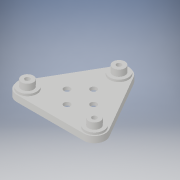
# Autodesk Inventor part: PlanetaryHolderTop
Saved by Autodesk Inventor 2018.3 (Build 223284000, 284)
## iProperties
Created: 2018-07-08
Part Number: PlanetaryHolderTop
Material: Generisch
Document SubType Name: Modeling
Designer: JochenAlt
Density: 1 g/cm^3
Appearance: Vorgabe
Author: JochenAlt
Autodesk Inventor part; units mm, degrees
ref_plane "YZ Plane" through (0, 0, 0) normal (1, 0, 0) x (0, 1, 0)
ref_plane "XZ Plane" through (0, 0, 0) normal (0, 1, 0) x (-1, 0, 0)
ref_plane "XY Plane" through (0, 0, 0) normal (0, 0, 1) x (1, 0, 0)
sketch "Skizze1" plane through (0, 0, 0) normal (0, 0, 1) x (1, 0, 0)
  circle A0 centre (0, 0) radius 18.538 construction
  circle A1 centre (0, 0) radius 9.75
  circle A2 centre (0, 18.538) radius 1.15
  line L0 (0, 0) -> (-16.0544, -9.269) construction
  line L1 (0, 32.8502) -> (0, -27.1027) construction
  line L2 (-31.8422, 0) -> (31.8422, 0) construction
  circle A3 centre (0, 0) radius 6.35 construction
  circle A4 centre (0, 6.35) radius 1.5
  circle A5 centre (0, -6.35) radius 1.5
  circle A6 centre (6.35, 0) radius 1.5
  circle A7 centre (-6.35, 0) radius 1.5
  arc A8 (0, 23.688) -> (-4.46, 21.113) centre (0, 18.538) ccw
  circle A9 centre (16.0544, -9.269) radius 1.15
  arc A10 (16.0544, -14.419) -> (20.5144, -6.694) centre (16.0544, -9.269) ccw
  circle A11 centre (-16.0544, -9.269) radius 1.15
  arc A12 (-20.5144, -6.694) -> (-16.0544, -14.419) centre (-16.0544, -9.269) ccw
  circle A13 centre (0, 18.538) radius 2.85
  circle A14 centre (16.0544, -9.269) radius 2.85
  circle A15 centre (-16.0544, -9.269) radius 2.85
  circle A16 centre (0, 18.538) radius 4.5
  circle A17 centre (16.0544, -9.269) radius 4.5
  circle A18 centre (-16.0544, -9.269) radius 4.5
  line L3 (-4.46, 21.113) -> (-20.5144, -6.694)
  line L4 (-16.0544, -14.419) -> (16.0544, -14.419)
  line L5 (4.46, 21.113) -> (20.5144, -6.694)
  arc A19 (4.46, 21.113) -> (0, 23.688) centre (0, 18.538) ccw
  circle A20 centre (0, 18.538) radius 2.1 construction
  line L6 (1.2124, 20.638) -> (2.4249, 18.538)
  line L7 (2.4249, 18.538) -> (1.2124, 16.438)
  line L8 (1.2124, 16.438) -> (-1.2124, 16.438)
  line L9 (-1.2124, 16.438) -> (-2.4249, 18.538)
  line L10 (-2.4249, 18.538) -> (-1.2124, 20.638)
  line L11 (-1.2124, 20.638) -> (1.2124, 20.638)
  circle A21 centre (-16.0544, -9.269) radius 2.1 construction
  circle A22 centre (16.0544, -9.269) radius 2.1 construction
  line L12 (-17.2654, -11.3698) -> (-18.4792, -9.2707)
  line L13 (-18.4792, -9.2707) -> (-17.2683, -7.1698)
  line L14 (-17.2683, -7.1698) -> (-14.8434, -7.1682)
  line L15 (-14.8434, -7.1682) -> (-13.6295, -9.2673)
  line L16 (-13.6295, -9.2673) -> (-14.8405, -11.3682)
  line L17 (-14.8405, -11.3682) -> (-17.2654, -11.3698)
  line L18 (15.1602, -11.523) -> (13.6553, -9.6216)
  line L19 (13.6553, -9.6216) -> (14.5494, -7.3676)
  line L20 (14.5494, -7.3676) -> (16.9485, -7.015)
  line L21 (16.9485, -7.015) -> (18.4535, -8.9164)
  line L22 (18.4535, -8.9164) -> (17.5593, -11.1704)
  line L23 (17.5593, -11.1704) -> (15.1602, -11.523)
  point P0 (0, 20.638)
  point P1 (-16.0544, -9.269)
  point P2 (-16.0529, -11.369)
  point P3 (16.3598, -11.3467)
  dimension "d31" = 4.2
  dimension "d0" = 37.076
  dimension "d1" = 2.3
  dimension "d2" = 30
  dimension "d3" = 19.5
  dimension "d4" = 12.7
  dimension "d5" = 3
  dimension "d8" = 4
  dimension "d26" = 5.7
  dimension "d30" = 9
  constraints: 44 end point, 20 centre point, 19 coincident, 16 point on circle, 12 equal radius, 7 point on line, 6 tangent, 3 midpoint, 1 concentric, 1 symmetric about line, 1 vertical alignment, 48 other
  measures "d0" diameter of A0
  measures "d1" diameter of A2
  measures "d2" angle of L0 L2
  measures "d3" diameter of A1
  measures "d4" diameter of A3
  measures "d5" diameter of A4
  measures "d8" radial gap between concentric circles of A2 A8
  measures "d26" diameter of A13
  measures "d30" diameter of A16
extrude "Extrusion1" add sketch "Skizze1" along normal blind 3 contours A1 | A19 L5 A10 L4 A12 L3 A8 | A13 | A14 | A15 | A16 | A17 | A18 | L6 L7 L8 L9 L10 L11 | L12 L13 L14 L15 L16 L17 | L18 L19 L20 L21 L22 L23
extrude "Extrusion3" cut sketch "Skizze1" along normal blind 1.5 contours A1
extrude "Extrusion4" add sketch "Skizze1" along normal blind 1 from surface at 3 contours A13 | A14 | A15 | A16 | A17 | A18 | L6 L7 L8 L9 L10 L11 | L12 L13 L14 L15 L16 L17 | L18 L19 L20 L21 L22 L23
extrude "Extrusion6" add sketch "Skizze1" along normal blind 3 from surface at 4 contours A13 | A14 | A15 | L6 L7 L8 L9 L10 L11 | L12 L13 L14 L15 L16 L17 | L18 L19 L20 L21 L22 L23
extrude "Extrusion8" cut sketch "Skizze1" along normal blind 1.5 contours L6 L7 L8 L9 L10 L11 | L12 L13 L14 L15 L16 L17 | L18 L19 L20 L21 L22 L23
